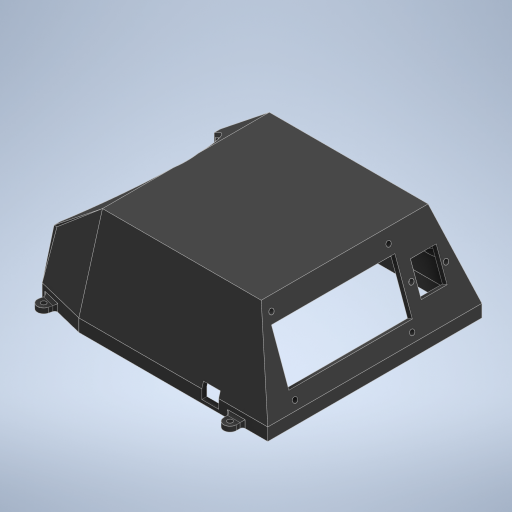
# Autodesk Inventor part: Base_Cover
Saved by Autodesk Inventor 2023 (Build 270158000, 158)
## iProperties
Created: 2024-08-01
Part Number: Base_Cover
Material: Generic
Document SubType Name: Modeling
Designer: Swoby
Density: 1 g/cm^3
Appearance: Default
Author: Swoby
Autodesk Inventor part; units mm, degrees
ref_plane "YZ Plane" through (0, 0, 0) normal (1, 0, 0) x (0, 1, 0)
ref_plane "XZ Plane" through (0, 0, 0) normal (0, 1, 0) x (-1, 0, 0)
ref_plane "XY Plane" through (0, 0, 0) normal (0, 0, 1) x (1, 0, 0)
sketch "Sketch1" plane through (0, 0, 0) normal (0, 1, 0) x (-1, 0, 0)
  line L0 (0, 85) -> (0, -85)
  line L1 (0, -85) -> (150, -85)
  line L2 (150, 85) -> (188.693081, 75.407162)
  line L3 (150, -85) -> (188.693081, -75.407162)
  arc A0 (232.502307, 64.545923) -> (209.491619, 66.129665) centre (216.5, 0) ccw construction
  line L4 (216.5, 0) -> (0, 0) construction
  line L5 (150, 85) -> (0, 85)
  line L6 (4, 81) -> (4, -81)
  line L7 (4, -81) -> (149.511551, -81)
  line L8 (149.511551, -81) -> (184.693081, -72.27775)
  line L9 (149.511551, 81) -> (4, 81)
  line L10 (209.491619, 66.129665) -> (188.693081, 71.286065) construction
  arc A1 (209.491619, 66.129665) -> (188.693081, 60.407162) centre (216.5, 0) ccw construction
  arc A2 (209.491619, -66.129665) -> (232.502307, -64.545923) centre (216.5, 0) ccw construction
  line L11 (188.693081, -75.407162) -> (188.693081, -60.407162)
  line L12 (188.693081, 60.407162) -> (188.693081, 75.407162)
  line L13 (184.693081, -76.398847) -> (184.693081, -72.27775) construction
  line L14 (184.693081, 58.400085) -> (184.693081, 72.27775)
  line L15 (188.693081, -75.407162) -> (232.502307, -64.545923) construction
  line L16 (188.693081, -71.286065) -> (209.491619, -66.129665) construction
  line L17 (184.693081, -72.27775) -> (184.693081, -58.400085)
  line L18 (184.693081, -72.27775) -> (188.693081, -71.286065) construction
  arc A3 (188.693081, -60.407162) -> (209.491619, -66.129665) centre (216.5, 0) ccw construction
  arc A4 (184.693081, -58.400085) -> (188.693081, -60.407162) centre (216.5, 0) ccw
  line L19 (188.693081, 71.286065) -> (184.693081, 72.27775) construction
  line L20 (188.693081, 75.407162) -> (232.502307, 64.545923) construction
  line L21 (184.693081, 72.27775) -> (149.511551, 81)
  line L22 (184.693081, 72.27775) -> (184.693081, 76.398847) construction
  arc A5 (188.693081, 60.407162) -> (184.693081, 58.400085) centre (216.5, 0) ccw
  arc A6 (184.693081, 58.400085) -> (184.693081, -58.400085) centre (216.5, 0) ccw construction
  dimension "d0" = 170
  dimension "d3" = 150
  dimension "d4" = 216.5
  dimension "d5" = 133
  dimension "d6" = 150
  dimension "d7" = 4
  dimension "d8" = 4
  dimension "d10" = 4
  dimension "d11" = 4
  dimension "d69" = 15
  dimension "d70" = 4
  dimension "d72" = 4
  constraints: 46 end point, 21 point on circle, 10 tangent, 7 centre point, 7 collinear, 4 point on line, 4 vertical, 2 horizontal, 1 coincident, 1 midpoint, 1 parallel, 1 perpendicular, 1 other
  measures "d0" distance of L0.start L0.end
  measures "d3" distance of L0.end L1.end
  measures "d4" distance from line of L0 L4.start
  measures "d5" diameter of A0
  measures "d6" distance of L2.start L0.start
  measures "d7" distance between parallel lines of L5 L9
  measures "d8" distance between parallel lines of L0 L6
  measures "d10" distance between parallel lines of L2 L10
  measures "d11" distance between parallel lines of L3 L8
  measures "d69" distance of L3.end L11.end
  measures "d70" distance between parallel lines of L17 L11
  measures "d72" distance between parallel lines of L2 L21
extrude "Extrusion1" add sketch "Sketch1" along normal blind 10
sketch "Sketch2" plane through (0, 0, 0) normal (0, -1, 0) x (1, 0, 0)
  circle A0 centre (-180.321642, 82.633991) radius 2
  arc A1 (-179.118461, 77.780914) -> (-175.468566, 83.837172) centre (-180.321642, 82.633991) ccw construction
  line L0 (0, 85) -> (0, -85)
  line L1 (-150, 85) -> (0, 85)
  line L2 (-188.693081, 75.407162) -> (-150, 85)
  line L3 (-4, 81) -> (-149.511551, 81)
  line L4 (-4, -81) -> (-4, 81)
  line L5 (-149.511551, -81) -> (-4, -81)
  line L6 (-184.693081, -72.27775) -> (-149.511551, -81)
  line L7 (-150, -85) -> (-188.693081, -75.407162)
  line L8 (0, -85) -> (-150, -85)
  line L9 (-185.174719, 81.43081) -> (-183.971538, 76.577733)
  line L10 (-175.468566, 83.837172) -> (-174.265385, 78.984095)
  circle A2 centre (-25, 90) radius 5
  circle A3 centre (-25, 90) radius 2
  line L11 (-25, 85) -> (-25, 90)
  line L12 (-30, 90) -> (-30, 85)
  line L13 (-20, 90) -> (-20, 85)
  line L14 (-30, 85) -> (-20, 85)
  arc A4 (-185.174719, 81.43081) -> (-179.118461, 77.780914) centre (-180.321642, 82.633991) ccw construction
  arc A5 (-175.468566, 83.837172) -> (-185.174719, 81.43081) centre (-180.321642, 82.633991) ccw
  line L15 (-180.321642, 82.633991) -> (-179.118461, 77.780914) construction
  line L16 (-188.693081, 60.407162) -> (-188.693081, 75.407162)
  arc A6 (-184.693081, 58.400085) -> (-188.693081, 60.407162) centre (-216.5, 0) ccw
  line L17 (-184.693081, 72.27775) -> (-184.693081, 58.400085)
  line L18 (-149.511551, 81) -> (-184.693081, 72.27775)
  line L19 (-184.693081, -58.400085) -> (-184.693081, -72.27775)
  arc A7 (-188.693081, -60.407162) -> (-184.693081, -58.400085) centre (-216.5, 0) ccw
  line L20 (-188.693081, -75.407162) -> (-188.693081, -60.407162)
  point P0 (0, 0)
  point P1 (-183.971538, 76.577733)
  point P2 (-174.265385, 78.984095)
  dimension "d14" = 4
  dimension "d15" = 10
  dimension "d16" = 25
  dimension "d17" = 10
  dimension "d18" = 4
  dimension "d19" = 5
  dimension "d66" = 30
  constraints: 14 end point, 8 point on circle, 7 tangent, 6 centre point, 3 coincident, 3 parallel, 2 perpendicular, 2 point on line, 1 collinear, 1 vertical
  measures "d14" diameter of A0
  measures "d15" diameter of A1
  measures "d16" distance of L0.start L11.start
  measures "d17" diameter of A2
  measures "d18" diameter of A3
  measures "d19" distance of L11.start L11.end
  measures "d66" distance of L1.start L15.end
extrude "Extrusion2" add sketch "Sketch2" against normal blind 4 contours L1 A2 L13 | L1 L12 A2 | A2 | L2 L9 A5 L10
mirror "Mirror1" about plane through (0, 0, 0) normal (0, 0, 1) of "Extrusion2"
fillet "Fillet1" radius 2 12 edges at (-183.9715, 2, -76.5777) (-179.1185, 4, -77.7809) (-174.2654, 2, -78.9841) (-30, 2, -85) (-25, 4, -85) (-20, 2, -85) (-20, 2, 85) (-25, 4, 85) (-174.2654, 2, 78.9841) (-179.1185, 4, 77.7809) (-30, 2, 85) (-183.9715, 2, 76.5777)
ref_plane "Work Plane1" through (0, 10, 85) normal (0.9396926, 0.3420201, 0) x (0, 0, -1)
sketch "Sketch3" plane through (0, 10, 85) normal (0.9396926, 0.3420201, 0) x (0, 0, -1)
  line L0 (0, 0) -> (170, 0)
  line L1 (0, 0) -> (18.756443, 70)
  line L2 (18.756443, 70) -> (151.243557, 70)
  line L3 (151.243557, 70) -> (170, 0)
  line L4 (21.256443, 13.15) -> (119.256443, 13.15)
  line L5 (119.256443, 13.15) -> (119.256443, 53.65)
  line L6 (119.256443, 53.65) -> (21.256443, 53.65)
  line L7 (21.256443, 53.65) -> (21.256443, 13.15)
  line L8 (20.756443, 63.8) -> (119.756443, 63.8)
  line L9 (119.756443, 63.8) -> (119.756443, 3)
  line L10 (119.756443, 3) -> (20.756443, 3)
  line L11 (20.756443, 3) -> (20.756443, 63.8)
  line L12 (128.993557, 46.05) -> (149.493557, 46.05)
  line L13 (149.493557, 46.05) -> (149.493557, 20.75)
  line L14 (149.493557, 20.75) -> (128.993557, 20.75)
  line L15 (128.993557, 20.75) -> (128.993557, 46.05)
  line L16 (128.993557, 33.4) -> (149.493557, 33.4) construction
  line L17 (139.243557, 46.05) -> (139.243557, 20.75) construction
  circle A0 centre (23.756443, 60.8) radius 2
  circle A1 centre (116.756443, 60.8) radius 2
  circle A2 centre (23.756443, 6) radius 2
  circle A3 centre (116.756443, 6) radius 2
  circle A4 centre (23.756443, 6) radius 4
  circle A5 centre (23.756443, 60.8) radius 4
  circle A6 centre (116.756443, 60.8) radius 4
  circle A7 centre (116.756443, 6) radius 4
  circle A8 centre (152.993557, 33.4) radius 2
  circle A9 centre (125.493557, 33.4) radius 2
  point P0 (85, -9.396926)
  point P1 (119.256443, 33.4)
  point P2 (119.756443, 3.354249)
  point P3 (119.402195, 3)
  point P4 (114.110692, 3)
  point P5 (26.402195, 3)
  point P6 (21.110692, 3)
  point P7 (20.756443, 3.354249)
  point P8 (20.756443, 8.645751)
  point P9 (20.756443, 58.154249)
  point P10 (20.756443, 63.445751)
  point P11 (21.110692, 63.8)
  point P12 (26.402195, 63.8)
  point P13 (114.110692, 63.8)
  point P14 (119.402195, 63.8)
  point P15 (119.756443, 63.445751)
  point P16 (119.756443, 58.154249)
  point P17 (119.756443, 8.645751)
  dimension "d24" = 75
  dimension "d25" = 75
  dimension "d26" = 70
  dimension "d27" = 98
  dimension "d28" = 40.5
  dimension "d29" = 99
  dimension "d30" = 0.5
  dimension "d31" = 60.8
  dimension "d32" = 10.15
  dimension "d33" = 3
  dimension "d34" = 2
  dimension "d35" = 20.5
  dimension "d36" = 25.3
  dimension "d38" = 4
  dimension "d39" = 4
  dimension "d40" = 4
  dimension "d41" = 4
  dimension "d42" = 1
  dimension "d43" = 1
  dimension "d44" = 1
  dimension "d46" = 1
  dimension "d48" = 1
  dimension "d49" = 1
  dimension "d50" = 1
  dimension "d51" = 1
  dimension "d52" = 8
  dimension "d53" = 8
  dimension "d54" = 8
  dimension "d55" = 8
  dimension "d93" = 4
  dimension "d94" = 4
  dimension "d95" = 3.5
  dimension "d96" = 3.5
  dimension "d97" = 12
  constraints: 34 end point, 10 centre point, 6 parallel, 5 midpoint, 4 coincident, 4 horizontal, 3 perpendicular, 3 point on line
  measures "d24" angle of L0 L1
  measures "d25" angle of L0 L3
  measures "d26" distance between parallel lines of L0 L2
  measures "d27" distance of L5.end L6.end
  measures "d28" distance of L4.end L5.end
  measures "d29" distance of L8.start L8.end
  measures "d30" distance between parallel lines of L7 L11
  measures "d31" distance between parallel lines of L10 L8
  measures "d32" distance between parallel lines of L6 L8
  measures "d33" distance between parallel lines of L0 L10
  measures "d34" distance from line of L1.end L11
  measures "d35" distance of L12.start L12.end
  measures "d36" distance of L14.end L12.start
  measures "d38" diameter of A0
  measures "d39" diameter of A1
  measures "d40" diameter of A2
  measures "d41" diameter of A3
  measures "d42" distance edge to line of A2 L10
  measures "d43" distance edge to line of A2 L11
  measures "d44" distance edge to line of A0 L11
  measures "d46" distance edge to line of A0 L8
  measures "d48" distance edge to line of A1 L8
  measures "d49" distance edge to line of A1 L9
  measures "d50" distance edge to line of A3 L9
  measures "d51" distance edge to line of A3 L10
  measures "d52" diameter of A4
  measures "d53" diameter of A5
  measures "d54" diameter of A6
  measures "d55" diameter of A7
  measures "d93" diameter of A8
  measures "d94" diameter of A9
  measures "d95" distance from line of L15 A9.centre
  measures "d96" distance from line of L13 A8.centre
  measures "d97" horizontal distance of L2.end L17.start
extrude "Extrusion3" add sketch "Sketch3" against normal blind 4 contours L1 L2 L3 L0 | L8 A5 L11 | A5 L8 | L8 A5 L11 | L11 A5 | L8 A6 L9 A7 L10 A4 L11 A5 | A6 L8 | L8 A6 L9 | A4 L10 L11 | L11 A4 | L8 L9 A6 | L9 A6 | A4 L10 L11 | A7 L9 | L9 A7 L10 | L10 A4 | L9 L10 A7 | L10 A7
extrude "Extrusion4" add sketch "Sketch3" against normal blind 7 contours A5 L8 | L8 A5 L11 | L11 A5 | A6 L8 | L8 A6 L9 | A4 L10 L11 | L11 A4 | L9 A6 | A7 L9 | L9 A7 L10 | L10 A4 | L10 A7 picked at (23.676085, 63.461806) picked at (116.836801, 63.461806) picked at (23.676085, 3.338194) picked at (116.836801, 3.338194)
ref_plane "Work Plane2" through (-150, 0, -85) normal (1, 0, 0) x (0, 1, 0)
sketch "Sketch5" plane through (-150, 0, -85) normal (1, 0, 0) x (0, 1, 0)
  line L0 (0, 0) -> (10, 0)
  line L1 (10, 0.390102) -> (10, 0)
  line L2 (10, 0) -> (10, 9.592838)
  line L3 (10, 12.72225) -> (10, 4)
  line L4 (10, 4) -> (10, 0.390102)
  line L5 (9.294692, 4) -> (10, 4)
  line L6 (0, 4) -> (10, 4)
  line L7 (0, 4) -> (9.294692, 4)
  line L8 (10, 166) -> (9.294692, 166)
  line L9 (0, 166) -> (9.294692, 166)
  line L10 (0, 166) -> (10, 166)
  line L11 (6, 170) -> (0, 170)
  line L12 (0, 170) -> (6, 170)
  line L13 (0, 170) -> (10, 170)
  line L14 (0, 170) -> (10, 170)
  line L15 (10, 170) -> (10, 169.609898)
  line L16 (75.778483, 151.243557) -> (10, 170)
  line L17 (75.778483, 151.243557) -> (74.410403, 151.243557)
  line L18 (10, 169.609898) -> (74.410403, 151.243557)
  line L19 (10, 0.390102) -> (10, 0)
  line L20 (74.410403, 18.756443) -> (10, 0.390102)
  line L21 (75.778483, 18.756443) -> (74.410403, 18.756443)
  line L22 (10, 0) -> (75.778483, 18.756443)
  line L23 (75.778483, 18.756443) -> (75.778483, 151.243557)
  line L24 (10, 4) -> (72.778483, 21.901007)
  line L25 (10, 166) -> (72.778483, 148.098993)
  line L26 (10, 166) -> (10, 170)
  line L27 (10, 9.592838) -> (10, 24.592838)
  line L28 (10, 24.592838) -> (10, 26.599915)
  line L29 (10, 26.599915) -> (10, 12.72225)
  line L30 (72.778483, 21.901007) -> (72.778483, 148.098993)
  point P0 (0, 85)
  dimension "d75" = 3
  constraints: 10 end point, 2 parallel, 2 vertical, 1 collinear
  measures "d75" distance between parallel lines of L30 L23
extrude "Extrusion6" add sketch "Sketch5" along normal up to surface surface through (-11.594483, 41.85558, 15.243557) normal (0.9396926, 0.3420201, 0)
ref_plane "Work Plane3" through (-188.693081, 0, -75.407162) normal (-0.9706154, 0, 0.2406362) x (0, 1, 0)
sketch "Sketch7" plane through (-188.693081, 0, -75.407162) normal (-0.9706154, 0, 0.2406362) x (0, 1, 0)
  line L0 (10, -161.122153) -> (72.778483, -143.747161)
  line L1 (10, -165.004615) -> (10, -161.122153)
  line L2 (75.778483, -146.799322) -> (10, -165.004615)
  line L3 (75.778483, -18.205293) -> (75.778483, -146.799322)
  line L4 (10, 0) -> (75.778483, -18.205293)
  line L5 (10, -3.882462) -> (10, 0)
  line L6 (72.778483, -21.257454) -> (10, -3.882462)
  line L7 (72.778483, -143.747161) -> (72.778483, -21.257454)
  line L8 (72.778483, -21.257454) -> (75.778483, -22.087754)
  point P0 (0, -118.597738)
  constraints: 2 end point, 1 collinear, 1 point on line
extrude "Extrusion8" add sketch "Sketch7" against normal up to surface contours L6 L5 L4 L3 L8 surface through (-150, 42.889242, 0) normal (1, 0, 0)
ref_plane "Work Plane4" through (-188.693081, 0, 75.407162) normal (0.9706154, 0, 0.2406362) x (0, 1, 0)
sketch "Sketch8" plane through (-188.693081, 0, 75.407162) normal (0.9706154, 0, 0.2406362) x (0, 1, 0)
  line L0 (75.778483, -142.916861) -> (72.778483, -143.747161)
  line L1 (72.778483, -21.257454) -> (72.778483, -143.747161)
  line L2 (10, -3.882462) -> (72.778483, -21.257454)
  line L3 (10, 0) -> (10, -3.882462)
  line L4 (75.778483, -18.205293) -> (10, 0)
  line L5 (75.778483, -142.916861) -> (75.778483, -18.205293)
  line L6 (72.778483, -21.257454) -> (75.778483, -22.087754)
  point P0 (0, -118.597738)
  constraints: 2 end point, 1 collinear, 1 point on line
extrude "Extrusion9" add sketch "Sketch8" along normal up to surface contours L6 L2 L3 L4 L5 surface through (-150, 42.889242, 0) normal (1, 0, 0)
sketch "Sketch9" plane through (-188.693081, 0, -75.407162) normal (-1, 0, 0) x (0, 0, 1)
  line L0 (0, 10) -> (15, 10)
  line L1 (17.670337, 75.778483) -> (0, 10)
  line L2 (135.814324, 10) -> (150.814324, 10)
  line L3 (133.143987, 75.778483) -> (150.814324, 10)
  line L4 (15, 10) -> (15, 45)
  line L5 (15, 45) -> (9.40219, 45)
  line L6 (135.814324, 10) -> (135.814324, 45)
  line L7 (135.814324, 45) -> (141.412134, 45)
  point P0 (75.407162, 0)
  dimension "d82" = 35
  constraints: 8 end point, 2 perpendicular, 2 point on line, 2 vertical, 1 collinear
  measures "d82" distance of L0.end L4.end
extrude "Extrusion10" add sketch "Sketch9" against normal up to surface (4 mm away)
ref_plane "Work Plane5" through (-150, 75.778483, -66.243557) normal (0.6225223, -0.7826021, 0) x (0, 0, 1)
sketch "Sketch10" plane through (-150, 75.778483, -66.243557) normal (0.6225223, -0.7826021, 0) x (0, 0, 1)
  line L0 (4, 0) -> (128.487113, 0)
  line L1 (5.836394, 49.441577) -> (0.238584, 49.441577)
  line L2 (132.248529, 49.441577) -> (126.650719, 49.441577)
  line L3 (5.836394, 49.441577) -> (126.650719, 49.441577)
  line L4 (0, 0) -> (0, -98.653714)
  line L5 (132.487113, 0) -> (132.487113, -98.653714)
  line L6 (0.238584, 49.441577) -> (0, 0)
  line L7 (4, 0) -> (0, 0)
  line L8 (128.487113, 0) -> (132.487113, 0)
  line L9 (132.487113, 0) -> (132.248529, 49.441577)
  point P0 (66.243557, -70.216516)
  constraints: 10 end point, 2 horizontal
extrude "Extrusion11" add sketch "Sketch10" along normal blind 3
sketch "Sketch11" plane through (-32, 0, -85) normal (0, 0, -1) x (-1, 0, 0)
  line L0 (118, 75.778483) -> (154.23168, 46.957926)
  line L1 (152.312228, 75.778483) -> (154.23168, 46.957926)
  line L2 (152.312228, 75.778483) -> (118, 75.778483)
  point P0 (-32, 0)
extrude "Extrusion12" cut sketch "Sketch11" against normal through all
sketch "Sketch12" plane through (0, 0, 0) normal (0, -1, 0) x (1, 0, 0)
  arc A0 (-188.693081, -60.407162) -> (-184.693081, -58.400085) centre (-216.5, 0) ccw
  arc A1 (-184.693081, 58.400085) -> (-188.693081, 60.407162) centre (-216.5, 0) ccw
  arc A2 (-184.693081, -58.400085) -> (-184.693081, 58.400085) centre (-216.5, 0) ccw construction
  arc A3 (-184.358271, 59.014822) -> (-188.693081, 61.176918) centre (-216.5, 0) ccw
  arc A4 (-184.358271, -59.014822) -> (-184.358271, 59.014822) centre (-216.5, 0) ccw
  arc A5 (-188.693081, -61.176918) -> (-184.358271, -59.014822) centre (-216.5, 0) ccw
  line L0 (-188.693081, -75.407162) -> (-188.693081, -60.407162)
  line L1 (-188.693081, 60.407162) -> (-188.693081, 75.407162)
  line L2 (-188.693081, -60.407162) -> (-188.693081, 60.407162)
  point P0 (0, 0)
  dimension "d89" = 0.7
  constraints: 8 point on circle, 4 centre point, 2 end point, 2 point on line, 1 collinear, 1 concentric
  measures "d89" radial gap between concentric circles of A2 A4
extrude "Extrusion13" cut sketch "Sketch12" against normal through all
sketch "Sketch13" plane through (-3.75877, 8.631919, 85) normal (-0.9396926, -0.3420201, 0) x (0, 0, 1)
  circle A0 centre (-152.993557, 33.4) radius 2
  circle A1 centre (-152.993557, 33.4) radius 2
  circle A2 centre (-152.993557, 33.4) radius 6.25
  point P0 (-85, -9.396926)
  dimension "d98" = 12.5
  constraints: 1 centre point, 1 coincident
  measures "d98" diameter of A2
extrude "Extrusion14" cut sketch "Sketch13" along normal through all
sketch "Sketch14" plane through (-4, 0, 81) normal (0, 0, -1) x (-1, 0, 0)
  line L0 (35, 2.7) -> (48.4, 2.7)
  line L1 (48.4, 2.7) -> (48.4, 14.7)
  line L2 (48.4, 14.7) -> (35, 14.7)
  line L3 (35, 14.7) -> (35, 2.7)
  line L4 (146, 0) -> (28, 0) projected
  line L5 (-4, 0) -> (-4, 10) projected
  dimension "d101" = 13.4
  dimension "d102" = 12
  dimension "d103" = 2.7
  dimension "d104" = 39
  constraints: 8 end point, 2 parallel, 1 horizontal, 1 perpendicular
  measures "d101" distance of L1.end L2.end
  measures "d102" distance of L0.end L1.end
  measures "d103" distance between parallel lines of L4 L0
  measures "d104" distance between parallel lines of L5 L3
extrude "Extrusion15" cut sketch "Sketch14" along normal mid plane 10
sketch "Sketch15" plane through (-149.511551, 0, -81) normal (0, 0, 1) x (1, 0, 0)
  circle A0 centre (95.511551, 4.5) radius 4.5
  line L0 (117.511551, 0) -> (-0.488449, 0)
  line L1 (91.011551, 4.5) -> (91.011551, 0)
  line L2 (100.011551, 4.5) -> (100.011551, 0)
  line L3 (149.511551, 0) -> (149.511551, 10)
  point P0 (95.511551, 0)
  dimension "d107" = 9
  dimension "d108" = 54
  constraints: 4 end point, 3 tangent, 2 perpendicular, 2 point on circle, 2 point on line, 1 centre point
  measures "d107" diameter of A0
  measures "d108" distance from line of L3 A0.centre
extrude "Extrusion16" cut sketch "Sketch15" against normal blind 10
equation "\"d19\" = 0.5 * d17"
equation "\"d25\" = d24"
equation "\"d30\" = -0.5 * d27 + 0.5 * d29"
equation "\"d32\" = -0.5 * d28 + 0.5 * d31"
equation "\"d43\" = d42"
equation "\"d44\" = d43"
equation "\"d46\" = d44"
equation "\"d48\" = d46"
equation "\"d50\" = d42"
equation "\"d51\" = d50"
body "Solid1"
